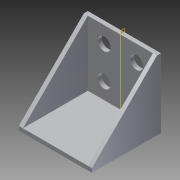
# Autodesk Inventor part: Milled Flange Support
Saved by Autodesk Inventor 2014 (Build 180170000, 170)
## iProperties
Created: 2014-01-05
Part Number: Milled Flange Support
Material: Aluminum 6061
Document SubType Name: Modeling
Designer: Michael
Density: 2.71 g/cm^3
Appearance: Aluminum - Flat
Author: Michael
Autodesk Inventor part; units mm, degrees
ref_plane "YZ Plane" through (0, 0, 0) normal (1, 0, 0) x (0, 1, 0)
ref_plane "XZ Plane" through (0, 0, 0) normal (0, 1, 0) x (-1, 0, 0)
ref_plane "XY Plane" through (0, 0, 0) normal (0, 0, 1) x (1, 0, 0)
sketch "Sketch1" plane through (0, 0, 0) normal (0, 0, 1) x (1, 0, 0)
  line L0 (0, 0) -> (25.4, 0)
  line L1 (25.4, 0) -> (25.4, 25.4)
  line L2 (25.4, 25.4) -> (0, 25.4)
  line L3 (0, 25.4) -> (0, 0)
  circle A0 centre (6.35, 19.05) radius 2.4892
  line L4 (12.7, 25.4) -> (12.7, 0) construction
  line L5 (0, 12.7) -> (25.4, 12.7) construction
  circle A1 centre (19.05, 19.05) radius 2.4892
  circle A2 centre (6.35, 6.35) radius 2.4892
  circle A3 centre (19.05, 6.35) radius 2.4892
  dimension "d0" = 25.4
  dimension "d1" = 25.4
  dimension "d2" = 4.9784
  dimension "d3" = 6.35
  dimension "d4" = 6.35
  constraints: 12 end point, 4 centre point, 4 midpoint, 3 symmetric about line, 2 parallel, 1 horizontal, 1 perpendicular, 3 other
  measures "d0" distance of L2.end L1.end
  measures "d1" distance of L1.end L0.end
  measures "d2" diameter of A0
  measures "d3" distance from line of L2 A0.centre
  measures "d4" distance from line of L3 A0.centre
extrude "Extrusion1" add sketch "Sketch1" along normal blind 1.5875
sketch "Sketch2" plane through (0, 0, 0) normal (-1, 0, 0) x (0, 0, 1)
  line L0 (0, 25.4) -> (0, 0) projected
  line L1 (0, 0) -> (1.5875, 0) projected
  line L2 (0, 25.4) -> (1.5875, 25.4) projected
  line L3 (1.5875, 25.4) -> (26.9875, 0)
  line L4 (1.5875, 25.4) -> (37.5085, 25.4) construction
  line L5 (26.9875, 0) -> (1.5875, 0)
  line L6 (1.5875, 25.4) -> (1.5875, 0)
  dimension "d7" = 45
  constraints: 8 end point, 1 equal length, 1 horizontal, 1 parallel, 1 perpendicular
  measures "d7" angle of L3 L4
extrude "Extrusion2" add sketch "Sketch2" along normal blind 1.5875
ref_plane "Work Plane1" through (12.7, 0, 0) normal (1, 0, 0) x (0, 0, -1)
mirror "Mirror1" about plane through (12.7, 0, 0) normal (1, 0, 0) of "Extrusion2"
sketch "Sketch3" plane through (0, 0, 1.5875) normal (0, -1, 0) x (1, 0, 0)
  line L0 (-1.5875, 25.4) -> (26.9875, 25.4)
  line L1 (26.9875, 25.4) -> (26.9875, -1.5875)
  line L2 (26.9875, -1.5875) -> (-1.5875, -1.5875)
  line L3 (-1.5875, -1.5875) -> (-1.5875, 25.4)
  point P0 (0, -1.5875)
  constraints: 8 end point, 2 parallel, 1 horizontal, 1 perpendicular
extrude "Extrusion3" add sketch "Sketch3" along normal blind 1.5875
equation "\"d4\" = d3"
body "Solid1"
